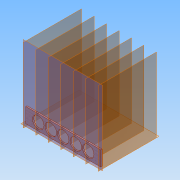
# Autodesk Inventor part: Timing_Base 1
Saved by Autodesk Inventor 2018.1 (Build 221171000, 171)
## iProperties
Created: 2019-02-11
Part Number: Timing_Base 1
Material: Wood (Oak)
Document SubType Name: Modeling
Designer: James
Density: 0.76 g/cm^3
Appearance: White Oak - Natural Medium Gloss
Author: James
Autodesk Inventor part; units mm, degrees
ref_plane "YZ Plane" through (0, 0, 0) normal (1, 0, 0) x (0, 1, 0)
ref_plane "XZ Plane" through (0, 0, 0) normal (0, 1, 0) x (-1, 0, 0)
ref_plane "XY Plane" through (0, 0, 0) normal (0, 0, 1) x (1, 0, 0)
derived "Selection_Skeleton.ipt"
ref_plane "Ground" through (0, 0, 0) normal (0, 1, 0) x (-1, 0, 0)
ref_plane "LHS inner" through (0, 0, 0) normal (1, 0, 0) x (0, 1, 0)
ref_plane "RHS inner" through (300, 0, 0) normal (1, 0, 0) x (0, 1, 0)
ref_plane "Lane 1" through (50, 0, 0) normal (1, 0, 0) x (0, 1, 0)
ref_plane "Lane 2" through (100, 0, 0) normal (1, 0, 0) x (0, 1, 0)
ref_plane "Lane 3" through (150, 0, 0) normal (1, 0, 0) x (0, 1, 0)
ref_plane "Lane 4" through (200, 0, 0) normal (1, 0, 0) x (0, 1, 0)
ref_plane "Lane 5" through (250, 0, 0) normal (1, 0, 0) x (0, 1, 0)
ref_plane "Back" through (0, 0, 0) normal (0, 0, 1) x (1, 0, 0)
sketch "Sketch1" plane through (0, 0, 0) normal (0, 1, 0) x (-1, 0, 0)
  line L0 (0, -12) -> (0, 72) projected
  line L1 (-300, -12) -> (-300, 72) projected
  line L2 (-360, 0) -> (60, 0) projected
  line L3 (0, 0) -> (-300, 0)
  line L4 (-300, 0) -> (-300, 60)
  line L5 (-300, 60) -> (0, 60)
  line L6 (0, 60) -> (0, 0)
  dimension "d1" = 60
  constraints: 8 end point, 2 parallel, 1 horizontal, 1 perpendicular, 1 point on line
  measures "d1" distance of L3.end L4.end
extrude "Extrusion1" add sketch "Sketch1" along normal blind 5
sketch "Sketch2" plane through (0, 5, 0) normal (0, 1, 0) x (1, 0, 0)
  line L0 (50, 12) -> (50, -72) projected
  line L1 (100, 12) -> (100, -72) projected
  line L2 (150, 12) -> (150, -72) projected
  line L3 (200, 12) -> (200, -72) projected
  line L4 (250, 12) -> (250, -72) projected
  line L5 (300, 0) -> (0, 0) projected
  line L6 (0, -60) -> (300, -60) projected
  point P0 (50, -30)
  dimension "d4" = 30
  dimension "d5" = 30
  constraints: 1 midpoint
  measures "d4" distance from line of point (50, -30) L5
  measures "d5" distance from line of L6 point (50, -30)
hole "Hole1" at (50, 5, 30) direction (0, -1, 0) diameter 46 end through all
pattern_linear "Rectangular Pattern1" count 5 spacing 50 along (1, 0, 0) of "Hole1"
equation "\"d4\" = d5"
body "Solid1"
